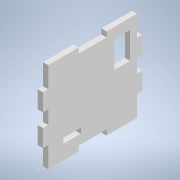
# Autodesk Inventor part: Lateral2
Saved by Autodesk Inventor 2020.2 (Build 242310000, 310)
## iProperties
Created: 2020-03-18
Part Number: Lateral2
Material: Generic
Document SubType Name: Modeling
Designer: ARQ SEVILLA R
Density: 1 g/cm^3
Appearance: Default
Author: ARQ SEVILLA R
Autodesk Inventor part; units mm, degrees
ref_plane "YZ Plane" through (0, 0, 0) normal (1, 0, 0) x (0, 1, 0)
ref_plane "XZ Plane" through (0, 0, 0) normal (0, 1, 0) x (-1, 0, 0)
ref_plane "XY Plane" through (0, 0, 0) normal (0, 0, 1) x (1, 0, 0)
sketch "Sketch1" plane through (0, 0, 0) normal (1, 0, 0) x (0, 1, 0)
  line L0 (0, -3) -> (12, -3)
  line L1 (12, -3) -> (12, 0)
  line L2 (12, 0) -> (22, 0)
  line L3 (22, 0) -> (22, -3)
  line L4 (25.875, 0) -> (25.875, -57) construction
  line L5 (51.75, -28.5) -> (0, -28.5) construction
  line L6 (51.75, -3) -> (39.75, -3)
  line L7 (39.75, -3) -> (39.75, 0)
  line L8 (39.75, 0) -> (29.75, 0)
  line L9 (29.75, 0) -> (29.75, -3)
  line L10 (12, 0) -> (22, 0)
  line L11 (29.75, 0) -> (39.75, 0)
  line L12 (39.75, 0) -> (29.75, 0)
  line L13 (22, 0) -> (12, 0)
  line L14 (22, -3) -> (29.75, -3)
  line L15 (0, -54) -> (12, -54)
  line L16 (12, -54) -> (12, -57)
  line L17 (12, -57) -> (22, -57)
  line L18 (22, -57) -> (22, -54)
  line L19 (51.75, -54) -> (39.75, -54)
  line L20 (29.75, -57) -> (29.75, -54)
  line L21 (39.75, -54) -> (39.75, -57)
  line L22 (39.75, -57) -> (29.75, -57)
  line L23 (22, -54) -> (29.75, -54)
  line L24 (39.75, -57) -> (29.75, -57)
  line L25 (22, -57) -> (12, -57)
  line L26 (0, -3) -> (0, -20.5)
  line L27 (0, -20.5) -> (3, -20.5)
  line L28 (3, -20.5) -> (3, -36.5)
  line L29 (3, -36.5) -> (0, -36.5)
  line L30 (0, -54) -> (0, -36.5)
  line L31 (51.75, -3) -> (51.75, -20.5)
  line L32 (51.75, -20.5) -> (48.75, -20.5)
  line L33 (48.75, -20.5) -> (48.75, -36.5)
  line L34 (48.75, -36.5) -> (51.75, -36.5)
  line L35 (51.75, -54) -> (51.75, -36.5)
  line L36 (0, -11.75) -> (8.25, -11.75) construction
  line L37 (8.25, -11.75) -> (8.25, -21.75)
  line L38 (8.25, -21.75) -> (11.25, -21.75)
  line L39 (11.25, -21.75) -> (11.25, -11.75)
  line L40 (11.25, -11.75) -> (8.25, -11.75)
  point P0 (0, 0)
  point P1 (51.75, 0)
  point P2 (0, 0)
  dimension "d0" = 51.75
  dimension "d2" = 3
  dimension "d3" = 12
  dimension "d4" = 10
  dimension "d5" = 17.5
  dimension "d6" = 3
  dimension "d7" = 16
  dimension "d8" = 8.25
  dimension "d9" = 10
  dimension "d10" = 3
  constraints: 82 end point, 20 symmetric about line, 8 perpendicular, 5 point on line, 4 horizontal, 1 midpoint
  measures "d0" distance of point (0, 0) point (51.75, 0)
  measures "d2" distance of L0.start point (0, 0)
  measures "d3" distance of L0.start L0.end
  measures "d4" distance of L2.end L1.end
  measures "d5" distance of L0.start L26.end
  measures "d6" distance of L26.end L27.end
  measures "d7" distance of L27.end L28.end
  measures "d8" distance of L36.start L36.end
  measures "d9" distance of L36.end L37.end
  measures "d10" distance of L37.end L38.end
extrude "Extrusion1" add sketch "Sketch1" along normal blind 3
sketch "Sketch2" plane through (3, 0, 0) normal (1, 0, 0) x (0, 0, -1)
  line L0 (54, 0) -> (54, 12) projected
  line L1 (50, 30.3502) -> (50, 45.7502)
  line L2 (50, 45.7502) -> (41, 45.7502)
  line L3 (41, 45.7502) -> (41, 30.3502)
  line L4 (41, 30.3502) -> (50, 30.3502)
  line L5 (54, 39.75) -> (54, 51.75) projected
  line L6 (54, 45.75) -> (50, 45.75)
  point P0 (0, 0)
  dimension "d15" = 15.4
  dimension "d16" = 9
  constraints: 10 end point, 2 perpendicular, 1 horizontal, 1 midpoint, 1 vertical
  measures "d15" distance of L1.start L1.end
  measures "d16" distance of L1.end L2.end
extrude "Extrusion2" cut sketch "Sketch2" against normal up to surface (3 mm away)
sketch "Sketch3" plane through (0, 0, 0) normal (-1, 0, 0) x (0, 0, 1)
  point P0 (0, 0)
body "Solid1"
